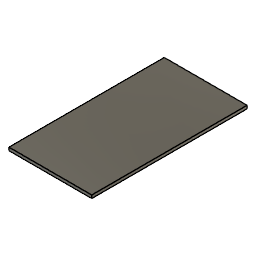
Drone Bellypack (Assembly) (Autodesk Fusion 360 archive; units mm, degrees)
design "Drone Bellypack"
part number: 2026-02-11-20-57-34-746
Autodesk Fusion 360 part; units mm, degrees
sketch "Sketch1" plane through (0, 0, 0) normal (0, 0, 1) x (1, 0, 0)
  line L0 (80, -150) -> (-80, -150)
  line L1 (-80, -150) -> (-80, 150)
  line L2 (-80, 150) -> (80, 150)
  line L3 (80, 150) -> (80, -150)
  line L4 (80, -150) -> (-80, 150) construction
  line L5 (-80, -150) -> (80, 150) construction
  dimension "d27" = 160
  dimension "d28" = 300
  constraint horizontal L0
  constraint perpendicular L0 L1
  constraint parallel L0 L2
  constraint parallel L1 L3
  constraint coincident L4 origin
  constraint coincident L5 origin
  measures "d27" distance of L1.end L2.end
  measures "d28" distance of L0.end L1.end
extrude "Extrude1" add sketch "Sketch1" along normal blind 6
sketch "Sketch2" plane through (0, 0, 6) normal (0, 0, 1) x (-1, 0, 0)
  line L0 (-80, -150) -> (80, -150)
  line L1 (80, -150) -> (80, 150)
  line L2 (80, 150) -> (-80, 150)
  line L3 (-80, 150) -> (-80, -150)
  circle A0 centre (66, 0) radius 6
  circle A1 centre (-66, 0) radius 6
  dimension "d31" = 12
  dimension "d32" = 12
  dimension "d33" = 132
  dimension "d34" = 66
  measures "d31" diameter of A0
  measures "d32" diameter of A1
  measures "d33" distance of A0.centre A1.centre
  measures "d34" distance of origin A0.centre
sketch "Sketch3" plane through (0, 0, 0) normal (0, 0, 1) x (1, 0, 0)
equation "tray_L = 300 mm"
equation "tray_W = 160 mm"
equation "tray_T = 6 mm"
equation "rail_d = 12 mm"
equation "rail_spacing = 132 mm"
equation "jet_L = 100 mm"
equation "jet_W = 80 mm"
equation "jet_H = 29 mm"
equation "spk_L = 84 mm"
equation "spk_W = 43 mm"
equation "spk_H = 32 mm"
equation "npf_L = 94 mm"
equation "npf_W = 47 mm"
equation "npf_H = 23 mm"
equation "buck = 62 mm"
equation "buck_W = 38 mm"
equation "buck_H = 14 mm"
equation "dd_L = 60 mm"
equation "dd_W = 33 mm"
equation "dd_H = 17 mm"
equation "mic_L = 14 mm"
equation "mic_W = 10 mm"
equation "mic_H = 3 mm"
equation "rad_L = 40 mm"
equation "rad_W = 40 mm"
equation "rad_H = 10 mm"
equation "d27 = tray_W"
equation "d28 = tray_L"
equation "d29 = tray_T"
equation "d31 = rail_d"
equation "d32 = rail_d"
equation "d33 = rail_spacing"
